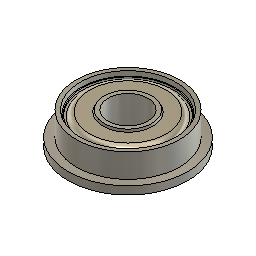
Spool Holder NG (Autodesk Fusion 360 archive; units mm, degrees)
design "F695 Bearing"
Autodesk Fusion 360 part; units mm, degrees
sketch "Sketch1" plane through (0, 0, 0) normal (0, 1, 0) x (1, 0, 0)
  circle A0 centre (0, 0) radius 7.5
  circle A1 centre (0, 0) radius 2.5
  dimension "d1" = 15
  dimension "d2" = 5
  constraint coincident A0.centre A1.centre
  constraint concentric A0 A1
  measures "d1" diameter of A0
  measures "d2" diameter of A1
extrude "Extrude1" add sketch "Sketch1" along normal blind 1
sketch "Sketch2" plane through (0, 1, 0) normal (0, 1, 0) x (-1, 0, 0)
  circle A0 centre (0, 0) radius 2.5
  circle A1 centre (0, 0) radius 7.5
  circle A2 centre (0, 0) radius 6.5
  dimension "d5" = 13
  constraint concentric A0 A2
  measures "d5" diameter of A2
extrude "Extrude2" add sketch "Sketch2" along normal blind 3 contours A2
sketch "Sketch3" plane through (0, 4, 0) normal (0, 1, 0) x (-1, 0, 0)
  circle A0 centre (0, 0) radius 2.5
  circle A1 centre (0, 0) radius 6.5
  circle A2 centre (0, 0) radius 3
  circle A3 centre (0, 0) radius 6
  circle A4 centre (0, 0) radius 3.125
  circle A5 centre (0, 0) radius 5.875
  circle A6 centre (0, 0) radius 5.5
  circle A7 centre (0, 0) radius 5.75
  dimension "d8" = 6
  dimension "d9" = 12
  dimension "d10" = 6.25
  dimension "d11" = 11.75
  dimension "d16" = 11
  dimension "d17" = 11.5
  constraint concentric A0 A2
  constraint concentric A2 A3
  constraint concentric A3 A4
  constraint concentric A4 A5
  constraint concentric A4 A6
  constraint concentric A6 A7
  measures "d8" diameter of A2
  measures "d9" diameter of A3
  measures "d10" diameter of A4
  measures "d11" diameter of A5
  measures "d16" diameter of A6
  measures "d17" diameter of A7
extrude "Extrude3" cut sketch "Sketch3" against normal blind 3 contours A3
extrude "Extrude4" cut sketch "Sketch3" against normal blind 3 contours A4
extrude "Extrude5" cut sketch "Sketch3" against normal blind 0.5 contours A5
extrude "Extrude6" cut sketch "Sketch3" against normal blind 0.75 contours A7
extrude "Extrude7" cut sketch "Sketch3" against normal blind 0.25 contours A6
fillet "Fillet1" radius 0.75 1 edges at (5.1278, 3.75, 1.9889)
sketch "Sketch4" plane through (0, 0, 0) normal (0, -1, 0) x (1, 0, 0)
  circle A0 centre (0, 0) radius 2.5
  circle A1 centre (0, 0) radius 7.5
  circle A2 centre (0, 0) radius 6
  circle A3 centre (0, 0) radius 3
  dimension "d25" = 12
  constraint concentric A0 A2
  constraint concentric A2 A3
  measures "d25" diameter of A2
extrude "Extrude8" cut sketch "Sketch4" against normal blind 0.25 contours A2
